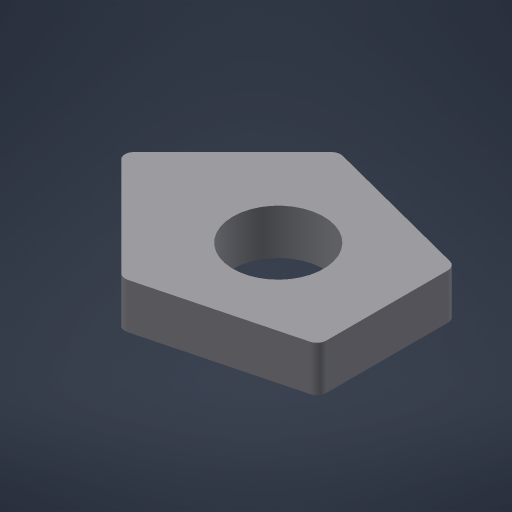
# Autodesk Inventor part: ALIGNMENT JIG 2SCREEN
Saved by Autodesk Inventor 2023.3 (Build 273359000, 359)
## iProperties
RuleStatus: InUse
Created: 2023-08-24
Material: Generic
Catalog Web Link: https://www.janelia.org/
Vendor: HHMI: JRC - jET
Document SubType Name: Modeling
Designer: jagers
Density: 1 g/cm^3
Appearance: Default
Part Number: ALIGNMENT JIG 2SCREEN
AfterDocSave0: file://Part Number Cleaner
DESIGN DEPARTMENT: HHMI: JRC - jET
ALTERED ITEM PART NUMBER: N/A
ALTERED ITEM VENDOR: N/A
ALTERED ITEM DESCRIPTION: N/A
Title: Standard
Author: jagers
Revision Number: 0
Autodesk Inventor part; units mm, degrees
ref_plane "YZ Plane" through (0, 0, 0) normal (1, 0, 0) x (0, 1, 0)
ref_plane "XZ Plane" through (0, 0, 0) normal (0, 1, 0) x (-1, 0, 0)
ref_plane "XY Plane" through (0, 0, 0) normal (0, 0, 1) x (1, 0, 0)
sketch "Sketch1" plane through (0, 0, 0) normal (0, 1, 0) x (-1, 0, 0)
  circle A0 centre (0, 0) radius 6.35
  line L0 (22, 0) -> (6.76, 15.24)
  line L1 (6.76, 15.24) -> (-15.24, 9.525)
  line L2 (-15.24, 9.525) -> (-15.24, 0)
  line L3 (22, 0) -> (0, 0)
  line L4 (22, 0) -> (6.76, -15.24)
  line L5 (6.76, -15.24) -> (-15.24, -9.525)
  line L6 (-15.24, -9.525) -> (-15.24, 0)
  dimension "d0" = 12.7
  dimension "d1" = 22
  dimension "d2" = 15.24
  dimension "d3" = 45
  dimension "d4" = 15.24
  dimension "d5" = 9.525
  constraints: 14 end point, 2 symmetric about line, 1 centre point, 1 coincident, 1 horizontal, 1 horizontal alignment, 1 vertical
  measures "d0" diameter of A0
  measures "d1" distance of L0.start L3.end
  measures "d2" distance from line of point (0, 0) L2
  measures "d3" angle of L3 L0
  measures "d4" distance from line of L3 L0.end
  measures "d5" distance of L1.end L2.end
extrude "Extrusion1" add sketch "Sketch1" along normal blind 6.35
fillet "Fillet1" radius 1.27 5 edges at (-22, 3.175, 0) (-6.76, 3.175, 15.24) (-6.76, 3.175, -15.24) (15.24, 3.175, 9.525) (15.24, 3.175, -9.525)
body "Solid1"
